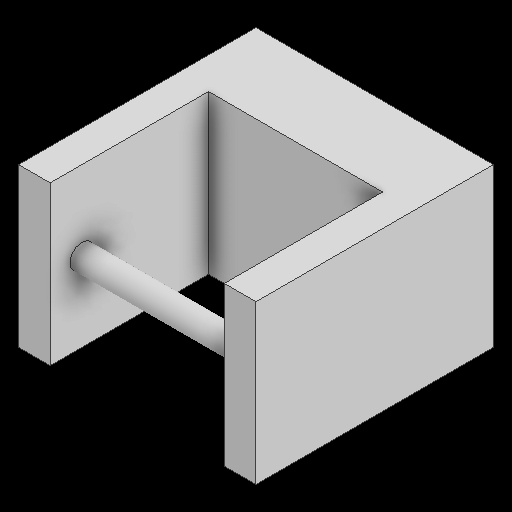
# Autodesk Inventor part: lever1
Saved by Autodesk Inventor 2025.1 (Build 291241000, 241)
## iProperties
Created: 2024-08-22
Part Number: lever1
Material: 일반
Document SubType Name: Modeling
Designer: ojs08
Density: 1 g/cm^3
Appearance: 기본값
Author: ojs08
Autodesk Inventor part; units mm, degrees
ref_plane "YZ Plane" through (0, 0, 0) normal (1, 0, 0) x (0, 1, 0)
ref_plane "XZ Plane" through (0, 0, 0) normal (0, 1, 0) x (-1, 0, 0)
ref_plane "XY Plane" through (0, 0, 0) normal (0, 0, 1) x (1, 0, 0)
sketch "스케치1" plane through (0, 0, 0) normal (0, 0, 1) x (1, 0, 0)
  line L0 (0, 0) -> (150, 0)
  line L1 (150, 0) -> (150, -100)
  line L2 (150, -100) -> (0, -100)
  line L3 (0, -100) -> (0, 0)
  dimension "d0" = 150
  dimension "d1" = 100
  constraints: 8 end point, 2 parallel, 1 coincident, 1 horizontal, 1 perpendicular
  measures "d0" distance of L0.start L0.end
  measures "d1" distance of L0.end L1.end
extrude "돌출1" add sketch "스케치1" along normal blind 50
sketch "스케치2" plane through (0, 0, 50) normal (0, 0, 1) x (1, 0, 0)
  line L0 (0, -100) -> (150, -100) projected
  line L1 (150, -100) -> (150, 0) projected
  line L2 (150, 0) -> (0, 0) projected
  line L3 (0, 0) -> (0, -100) projected
  line L4 (20, 0) -> (20, -100)
  line L5 (130, 0) -> (130, -100)
  dimension "d4" = 20
  dimension "d5" = 20
  constraints: 4 end point, 4 point on line, 2 perpendicular
  measures "d4" distance between parallel lines of L3 L4
  measures "d5" distance between parallel lines of L1 L5
extrude "돌출2" add sketch "스케치2" along normal blind 100 contours L3 L2 L4 L0 | L5 L2 L1 L0
sketch "스케치3" plane through (20, -100, 50) normal (1, 0, 0) x (0, 0, -1)
  line L0 (0, 100) -> (0, 0) projected
  line L1 (0, 100) -> (-100, 100) projected
  line L2 (-100, 0) -> (-100, 100) projected
  line L3 (0, 0) -> (-100, 0) projected
  circle A0 centre (-80, 50) radius 7.5
  point P0 (50, 100)
  dimension "d8" = 15
  dimension "d9" = 20
  dimension "d10" = 50
  constraints: 1 centre point
  measures "d8" diameter of A0
  measures "d9" distance from line of L2 A0.centre
  measures "d10" distance from line of L1 A0.centre
extrude "돌출3" add sketch "스케치3" along normal up to surface (110 mm away) contours A0
